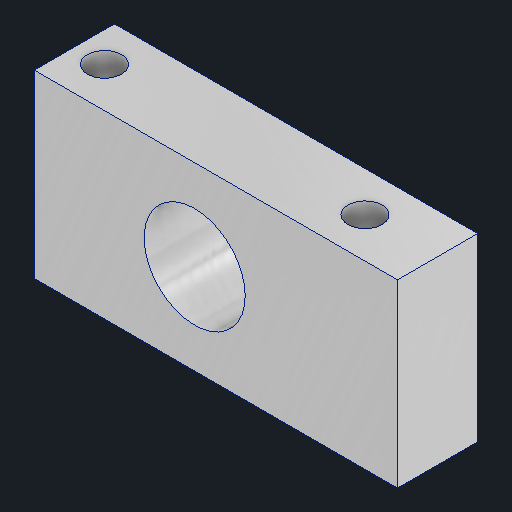
# Autodesk Inventor part: Drive Frame Tension Bearing Plate
Saved by Autodesk Inventor 2025.1 (Build 291241020, 241B)
## iProperties
Created: 2025-04-26
Part Number: Drive Frame Tension Bearing Plate
Material: Aluminum 6061
Document SubType Name: Modeling
Designer: Joshua Eah
Density: 2.7 g/cm^3
Appearance: Aluminum - Flat
Mass: 11.4803 g
Surface Area: 26.1468 cm^2
Volume: 4.25198 cm^3
Author: Joshua Eah
Autodesk Inventor part; units mm, degrees
ref_plane "YZ Plane" through (0, 0, 0) normal (1, 0, 0) x (0, 1, 0)
ref_plane "XZ Plane" through (0, 0, 0) normal (0, 1, 0) x (-1, 0, 0)
ref_plane "XY Plane" through (0, 0, 0) normal (0, 0, 1) x (1, 0, 0)
sketch "Sketch1" plane through (0, 0, 0) normal (0, 1, 0) x (-1, 0, 0)
  line L0 (0, 0) -> (-32, 0)
  line L1 (-32, 0) -> (-32, -8)
  line L2 (-32, -8) -> (0, -8)
  line L3 (0, -8) -> (0, 0)
  line L4 (0, -4) -> (-32, -4) construction
  circle A0 centre (-3, -4) radius 1.5
  circle A1 centre (-29, -4) radius 1.5
  dimension "d1" = 8
  dimension "d2" = 26
  dimension "d20" = 3
  dimension "d21" = 3
  dimension "d22" = 3
  constraints: 10 end point, 2 centre point, 2 midpoint, 2 parallel, 2 point on line, 1 equal radius, 1 horizontal, 1 perpendicular
  measures "d1" distance of L1.end L0.end
  measures "d2" distance of A0.centre A1.centre
  measures "d20" distance from line of A0.centre L3
  measures "d21" diameter of A0
  measures "d22" distance from line of L1 A1.centre
extrude "Extrusion1" add sketch "Sketch1" along normal blind 18 contours L3 L2 L1 L0 | A0 | A1
hole "Hole1" at (29, 0, -4) at (3, 0, -4) direction (0, 1, 0) diameter 3.4036 end through all clearance for "Flat Head Machine Screw" size "M3" standard "Ansi Metric M Profile"
sketch "Sketch2" plane through (0, 0, 0) normal (0, 0, 1) x (1, 0, 0)
  line L0 (0, 0) -> (32, 0) projected
  line L1 (32, 0) -> (32, 18) projected
  line L2 (0, 18) -> (32, 18) projected
  line L3 (0, 0) -> (0, 18) projected
  line L4 (0, 9) -> (32, 9)
  line L5 (32, 0) -> (32, 18) projected
  line L6 (16, 18) -> (16, 0)
  circle A0 centre (16, 9) radius 4.7625
  dimension "d28" = 9.525
  constraints: 5 midpoint, 4 end point, 1 centre point
  measures "d28" diameter of A0
hole "Hole2" at (16, 9, 0) direction (0, 0, -1) diameter 10.0838 end through all clearance for "Flat Head Machine Screw (82)" size "3/8" standard "Ansi Unified Screw Threads"
sketch "Sketch3" plane through (32, 0, 0) normal (1, 0, 0) x (0, 0, -1)
  line L0 (0, 0) -> (8, 0) projected
  line L1 (8, 0) -> (8, 18) projected
  line L2 (0, 18) -> (8, 18) projected
  line L3 (0, 0) -> (0, 18) projected
  point P0 (0, 0)
extrude "Extrusion2" add sketch "Sketch3" along normal blind 4.239
equation "\"d22\" = d20"
body "Solid1"
